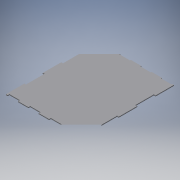
# Autodesk Inventor part: traseira
Saved by Autodesk Inventor 2016 (Build 200138000, 138)
## iProperties
Created: 2017-06-06
Part Number: traseira
Material: Genérico
Document SubType Name: Modeling
Designer: Fabio
Density: 1 g/cm^3
Appearance: Padrão
Author: Fabio
Autodesk Inventor part; units mm, degrees
ref_plane "YZ Plane" through (0, 0, 0) normal (1, 0, 0) x (0, 1, 0)
ref_plane "XZ Plane" through (0, 0, 0) normal (0, 1, 0) x (-1, 0, 0)
ref_plane "XY Plane" through (0, 0, 0) normal (0, 0, 1) x (1, 0, 0)
sketch "Esboço1" plane through (0, 0, 0) normal (0, 0, 1) x (1, 0, 0)
  line L0 (-173, 210) -> (173, 210)
  line L1 (173, 210) -> (173, -210)
  line L2 (173, -210) -> (-173, -210)
  line L3 (-173, -210) -> (-173, 210)
  point P0 (0, 0)
  point P1 (173, 0)
  point P2 (0, 210)
  dimension "d0" = 420
  dimension "d1" = 346
  constraints: 8 end point, 2 midpoint, 2 parallel, 1 horizontal, 1 horizontal alignment, 1 perpendicular, 1 vertical alignment
  measures "d0" distance between parallel lines of L0 L2
  measures "d1" distance between parallel lines of L3 L1
extrude "Extrusão1" add sketch "Esboço1" along normal blind 4
sketch "Esboço2" plane through (0, 0, 4) normal (0, 0, 1) x (1, 0, 0)
  line L0 (-173, 210) -> (-173, -210) projected
  line L1 (-173, -210) -> (173, -210) projected
  line L2 (-165, -202) -> (-118.5, -202)
  line L3 (-118.5, -202) -> (-118.5, -210)
  line L4 (-118.5, -210) -> (-165, -210)
  line L5 (-70.5, -210) -> (-24, -210)
  line L6 (-24, -210) -> (-24, -202)
  line L7 (-24, -202) -> (-70.5, -202)
  line L8 (-70.5, -202) -> (-70.5, -210)
  line L9 (24, -210) -> (70.5, -210)
  line L10 (70.5, -210) -> (70.5, -202)
  line L11 (70.5, -202) -> (24, -202)
  line L12 (24, -202) -> (24, -210)
  line L13 (118.5, -210) -> (165, -210)
  line L14 (165, -210) -> (165, -202)
  line L15 (165, -202) -> (118.5, -202)
  line L16 (118.5, -202) -> (118.5, -210)
  circle A0 centre (-118.5, -202) radius 1
  circle A1 centre (-70.5, -202) radius 1
  circle A2 centre (-24, -202) radius 1
  circle A3 centre (24, -202) radius 1
  circle A4 centre (70.5, -202) radius 1
  circle A5 centre (118.5, -202) radius 1
  line L17 (173, -210) -> (173, 210) projected
  line L18 (-165, -202) -> (-165, -210)
  circle A6 centre (165, -202) radius 1
  circle A7 centre (-165, -202) radius 1
  point P0 (0, 0)
  dimension "d4" = 46.5
  dimension "d5" = 8
  dimension "d6" = 46.5
  dimension "d7" = 46.5
  dimension "d8" = 46.5
  dimension "d9" = 8
  dimension "d10" = 8
  dimension "d11" = 48
  dimension "d12" = 48
  dimension "d13" = 48
  dimension "d16" = 2
  dimension "d17" = 2
  dimension "d18" = 2
  dimension "d19" = 2
  dimension "d20" = 2
  dimension "d21" = 2
  dimension "d38" = 8
  dimension "d40" = 46.5
  dimension "d41" = 2
  dimension "d42" = 2
  constraints: 32 end point, 8 centre point, 8 coincident, 7 parallel, 5 point on line, 4 horizontal, 4 perpendicular
  measures "d4" distance of L3.end L4.end
  measures "d5" distance between parallel lines of L1 L2
  measures "d6" distance of L7.end L6.end
  measures "d7" distance of L11.end L10.end
  measures "d8" distance of L15.end L14.end
  measures "d9" distance between parallel lines of L1 L7
  measures "d10" distance between parallel lines of L13 L15
  measures "d11" distance from line of L7.end L3
  measures "d12" distance between parallel lines of L12 L6
  measures "d13" distance between parallel lines of L16 L10
  measures "d16" diameter of A0
  measures "d17" diameter of A1
  measures "d18" diameter of A2
  measures "d19" diameter of A3
  measures "d20" diameter of A4
  measures "d21" diameter of A5
  measures "d38" distance between parallel lines of L17 L14
  measures "d40" distance of L2.start L2.end
  measures "d41" diameter of A6
  measures "d42" diameter of A7
extrude "Extrusão2" cut sketch "Esboço2" against normal blind 10
sketch "Esboço3" plane through (0, 0, 0) normal (0, 0, -1) x (-1, 0, 0)
  line L0 (-173, 210) -> (173, 210) projected
  line L1 (-118.5, 210) -> (-118.5, 206)
  line L2 (-118.5, 206) -> (-165, 206)
  line L3 (-70.5, 210) -> (-24, 210)
  line L4 (-24, 210) -> (-24, 206)
  line L5 (-24, 206) -> (-70.5, 206)
  line L6 (-70.5, 206) -> (-70.5, 210)
  line L7 (173, -210) -> (173, 210) projected
  circle A0 centre (-118.5, 206) radius 1
  circle A1 centre (-70.5, 206) radius 1
  circle A2 centre (-24, 206) radius 1
  line L8 (-165, 206) -> (-165, 210)
  line L9 (-118.5, 210) -> (-165, 210)
  line L10 (173, 210) -> (-173, 210) projected
  line L11 (-173, 210) -> (-173, -210) projected
  circle A3 centre (-165, 206) radius 1
  point P0 (0, 0)
  point P1 (173, -202)
  dimension "d22" = 46.5
  dimension "d23" = 4
  dimension "d24" = 46.5
  dimension "d31" = 48
  dimension "d33" = 2
  dimension "d34" = 2
  dimension "d35" = 2
  dimension "d43" = 8
  dimension "d44" = 2
  constraints: 16 end point, 4 centre point, 4 coincident, 2 parallel, 2 perpendicular, 2 point on line, 1 collinear, 1 horizontal
  measures "d22" distance of L1.end L2.end
  measures "d23" distance between parallel lines of L0 L2
  measures "d24" distance of L4.end L5.end
  measures "d31" horizontal distance of L5.end L1.start
  measures "d33" diameter of A0
  measures "d34" diameter of A1
  measures "d35" diameter of A2
  measures "d43" distance between parallel lines of L11 L8
  measures "d44" diameter of A3
extrude "Extrusão3" cut sketch "Esboço3" against normal blind 10
mirror "Espelhamento1" about plane through (0, 0, 0) normal (1, 0, 0) of "Extrusão3"
sketch "Esboço4" plane through (0, 0, 0) normal (0, 0, -1) x (-1, 0, 0)
  line L0 (173.5526, -126) -> (165.5526, -126)
  line L1 (165.5526, -126) -> (165.5526, -42)
  line L2 (165.5526, -42) -> (173.5526, -42)
  line L3 (173.5526, -42) -> (173.5526, -126)
  line L4 (165, -210) -> (173, -210) projected
  line L5 (173, 210) -> (173, -210) projected
  line L6 (173, 42) -> (165, 42)
  line L7 (165, 42) -> (165, 126)
  line L8 (165, 126) -> (173, 126)
  line L9 (173, 126) -> (173, 42)
  line L10 (173, 210) -> (165, 210) projected
  circle A0 centre (165.5526, -42) radius 1
  circle A1 centre (165.5526, -126) radius 1
  circle A2 centre (165, 42) radius 1
  circle A3 centre (165, 126) radius 1
  point P0 (0, 0)
  dimension "d45" = 8
  dimension "d46" = 84
  dimension "d47" = 84
  dimension "d48" = 84
  dimension "d49" = 84
  dimension "d50" = 84
  dimension "d51" = 2
  dimension "d52" = 2
  dimension "d53" = 2
  dimension "d54" = 2
  constraints: 16 end point, 4 centre point, 4 coincident, 4 parallel, 2 horizontal, 2 perpendicular, 1 point on line
  measures "d45" distance of L1.end L2.end
  measures "d46" distance between parallel lines of L2 L0
  measures "d47" distance between parallel lines of L4 L0
  measures "d48" distance between parallel lines of L6 L8
  measures "d49" distance between parallel lines of L2 L6
  measures "d50" distance between parallel lines of L10 L8
  measures "d51" diameter of A0
  measures "d52" diameter of A1
  measures "d53" diameter of A2
  measures "d54" diameter of A3
extrude "Extrusão4" cut sketch "Esboço4" against normal blind 10
mirror "Espelhamento2" about plane through (0, 0, 0) normal (1, 0, 0) of "Extrusão4"
